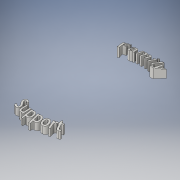
# Autodesk Inventor part: Team Pin Family-Text
Saved by Autodesk Inventor 2016 (Build 200138000, 138)
## iProperties
Created: 2016-02-20
Part Number: Team Pin Family-Text
Material: Generic
Document SubType Name: Modeling
Designer: RoksBot
Density: 1 g/cm^3
Appearance: White
Author: RoksBot
Autodesk Inventor part; units mm, degrees
ref_plane "YZ Plane" through (0, 0, 0) normal (1, 0, 0) x (0, 1, 0)
ref_plane "XZ Plane" through (0, 0, 0) normal (0, 1, 0) x (-1, 0, 0)
ref_plane "XY Plane" through (0, 0, 0) normal (0, 0, 1) x (1, 0, 0)
sketch "Sketch1" plane through (0, 0, 0) normal (0, 0, 1) x (1, 0, 0)
  line L0 (0, 0) -> (0, 8.6646) construction
  line L1 (20.9931, 1.27) -> (20.9931, 5.715)
  line L2 (20.9931, 5.715) -> (27.9781, 3.81)
  line L3 (27.9781, 3.81) -> (27.9781, 0)
  line L4 (27.9781, 0) -> (20.9931, 0)
  line L5 (20.9931, 1.27) -> (18.4531, 1.27)
  line L6 (18.4531, 1.27) -> (18.4531, 0)
  line L7 (18.4531, 0) -> (20.9931, 0)
  dimension "d0" = 20.9931
  dimension "d1" = 4.445
  dimension "d2" = 1.27
  dimension "d3" = 2.54
  dimension "d4" = 3.81
  dimension "d5" = 6.985
  constraints: 16 end point, 2 parallel, 2 perpendicular, 2 vertical, 1 horizontal, 1 horizontal alignment
  measures "d0" distance between parallel lines of L0 L1
  measures "d1" distance from line of L5 L1.end
  measures "d2" distance of L5.end L6.end
  measures "d3" distance between parallel lines of L1 L6
  measures "d4" distance of L2.end L3.end
  measures "d5" distance between parallel lines of L1 L3
revolve "Revolution1" add sketch "Sketch1" angle 360 about axis through (0, 0, 0) along (0, 1, 0)
sketch "Sketch2" plane through (0, 1.27, 0) normal (0, 1, 0) x (1, 0, 0)
  circle A0 centre (0, 0) radius 20.9931 projected
  circle A1 centre (0, 0) radius 27.9781 projected
  circle A2 centre (0, 0) radius 18.4531 projected
  circle A3 centre (0, 0) radius 20.9931 projected
  line L0 (-9.3205, 24.5047) -> (-8.9754, 23.5356)
  line L1 (-8.9754, 23.5356) -> (-7.525, 24.052)
  line L2 (-7.525, 24.052) -> (-7.3036, 23.43)
  line L3 (-7.3036, 23.43) -> (-8.754, 22.9135)
  line L4 (-8.754, 22.9135) -> (-8.0814, 21.0244)
  line L5 (-8.0814, 21.0244) -> (-8.8147, 20.7633)
  line L6 (-8.8147, 20.7633) -> (-10.2859, 24.8952)
  line L7 (-10.2859, 24.8952) -> (-7.5651, 25.8638)
  line L8 (-7.5651, 25.8638) -> (-7.3332, 25.2123)
  line L9 (-7.3332, 25.2123) -> (-9.3205, 24.5047)
  spline S0 degree 2 poles (-3.7722, 22.5301) (-3.8396, 22.3472) (-4.2977, 22.043) (-4.5708, 21.9904) knots 0 0 0 1 2 2 2
  spline S1 degree 2 poles (-4.5708, 21.9904) (-5.0792, 21.8924) (-5.7608, 22.2884) (-5.8502, 22.7525) knots 0 0 0 1 2 2 2
  spline S2 degree 2 poles (-5.8502, 22.7525) (-5.9554, 23.2985) (-5.2521, 24.0747) (-4.4979, 24.2201) knots 0 0 0 1 2 2 2
  spline S3 degree 2 poles (-4.4979, 24.2201) (-4.3682, 24.2451) (-4.1822, 24.2349) knots 0 0 0 1 1 1
  spline S4 degree 2 poles (-4.1822, 24.2349) (-4.2894, 24.7911) (-4.9924, 24.6557) knots 0 0 0 1 1 1
  spline S5 degree 2 poles (-4.9924, 24.6557) (-5.4087, 24.5754) (-5.6588, 24.3856) knots 0 0 0 1 1 1
  line L10 (-5.6588, 24.3856) -> (-5.9291, 24.9246)
  spline S6 degree 2 poles (-5.9291, 24.9246) (-5.5851, 25.1785) (-5.0596, 25.2798) knots 0 0 0 1 1 1
  spline S7 degree 2 poles (-5.0596, 25.2798) (-4.3395, 25.4186) (-3.5444, 24.8922) (-3.3688, 23.9811) knots 0 0 0 1 2 2 2
  line L11 (-3.3688, 23.9811) -> (-3.2386, 23.3054)
  spline S8 degree 2 poles (-3.2386, 23.3054) (-3.1176, 22.6775) (-2.8341, 22.5658) knots 0 0 0 1 1 1
  spline S9 degree 2 poles (-2.8341, 22.5658) (-2.896, 22.391) (-3.1033, 22.2732) (-3.2467, 22.2456) knots 0 0 0 1 2 2 2
  spline S10 degree 2 poles (-3.2467, 22.2456) (-3.4037, 22.2153) (-3.7016, 22.4021) (-3.7722, 22.5301) knots 0 0 0 1 2 2 2
  spline S11 degree 2 poles (-4.0682, 23.68) (-4.2631, 23.6813) (-4.3586, 23.6629) knots 0 0 0 1 1 1
  spline S12 degree 2 poles (-4.3586, 23.6629) (-5.2323, 23.4945) (-5.1231, 22.928) knots 0 0 0 1 1 1
  spline S13 degree 2 poles (-5.1231, 22.928) (-5.0415, 22.5049) (-4.5501, 22.5996) knots 0 0 0 1 1 1
  spline S14 degree 2 poles (-4.5501, 22.5996) (-3.8847, 22.7278) (-4.0116, 23.3865) knots 0 0 0 1 1 1
  line L12 (-4.0116, 23.3865) -> (-4.0682, 23.68)
  line L13 (1.4465, 22.5193) -> (1.4434, 24.5246)
  spline S15 degree 2 poles (1.4434, 24.5246) (1.4425, 25.1571) (0.876, 25.1563) knots 0 0 0 1 1 1
  spline S16 degree 2 poles (0.876, 25.1563) (0.7092, 25.156) (0.3967, 24.9574) (0.3343, 24.8288) knots 0 0 0 1 2 2 2
  line L14 (0.3343, 24.8288) -> (0.3378, 22.5176)
  line L15 (0.3378, 22.5176) -> (-0.4094, 22.5165)
  line L16 (-0.4094, 22.5165) -> (-0.4126, 24.64)
  spline S17 degree 2 poles (-0.4126, 24.64) (-0.4129, 24.8763) (-0.7053, 25.1539) (-0.9729, 25.1535) knots 0 0 0 1 2 2 2
  spline S18 degree 2 poles (-0.9729, 25.1535) (-1.1154, 25.1533) (-1.4452, 24.9442) (-1.5215, 24.819) knots 0 0 0 1 2 2 2
  line L17 (-1.5215, 24.819) -> (-1.518, 22.5148)
  line L18 (-1.518, 22.5148) -> (-2.2652, 22.5137)
  line L19 (-2.2652, 22.5137) -> (-2.2701, 25.718)
  line L20 (-2.2701, 25.718) -> (-1.7557, 25.7188)
  line L21 (-1.7557, 25.7188) -> (-1.6024, 25.4375)
  spline S19 degree 2 poles (-1.6024, 25.4375) (-1.2901, 25.7786) (-0.7966, 25.7793) knots 0 0 0 1 1 1
  spline S20 degree 2 poles (-0.7966, 25.7793) (-0.1606, 25.7803) (0.1631, 25.4332) knots 0 0 0 1 1 1
  spline S21 degree 2 poles (0.1631, 25.4332) (0.3054, 25.5933) (0.8056, 25.7817) (1.0593, 25.7821) knots 0 0 0 1 2 2 2
  spline S22 degree 2 poles (1.0593, 25.7821) (1.5945, 25.7829) (2.1897, 25.1721) (2.1905, 24.6369) knots 0 0 0 1 2 2 2
  line L22 (2.1905, 24.6369) -> (2.1937, 22.5204)
  line L23 (2.1937, 22.5204) -> (1.4465, 22.5193)
  line L24 (3.1822, 22.2932) -> (3.5833, 24.8512)
  line L25 (3.5833, 24.8512) -> (3.1781, 24.9147)
  line L26 (3.1781, 24.9147) -> (3.2734, 25.5224)
  line L27 (3.2734, 25.5224) -> (4.427, 25.3415)
  line L28 (4.427, 25.3415) -> (3.9307, 22.1759)
  line L29 (3.9307, 22.1759) -> (3.1822, 22.2932)
  spline S23 degree 2 poles (4.2524, 26.6283) (4.4309, 26.6003) (4.6423, 26.3103) (4.6143, 26.1318) knots 0 0 0 1 2 2 2
  spline S24 degree 2 poles (4.6143, 26.1318) (4.5863, 25.9533) (4.2963, 25.7419) (4.1178, 25.7699) knots 0 0 0 1 2 2 2
  spline S25 degree 2 poles (4.1178, 25.7699) (3.9393, 25.7979) (3.7279, 26.0879) (3.7559, 26.2664) knots 0 0 0 1 2 2 2
  spline S26 degree 2 poles (3.7559, 26.2664) (3.7839, 26.4449) (4.0739, 26.6563) (4.2524, 26.6283) knots 0 0 0 1 2 2 2
  line L30 (5.9373, 26.2566) -> (6.706, 26.2574)
  line L31 (6.706, 26.2574) -> (5.8627, 22.7535)
  spline S27 degree 2 poles (5.8627, 22.7535) (5.7244, 22.1791) (6.0422, 21.9847) knots 0 0 0 1 1 1
  spline S28 degree 2 poles (6.0422, 21.9847) (5.796, 21.7043) (5.3872, 21.8027) knots 0 0 0 1 1 1
  spline S29 degree 2 poles (5.3872, 21.8027) (4.8939, 21.9215) (5.0589, 22.6074) knots 0 0 0 1 1 1
  line L32 (5.0589, 22.6074) -> (5.9373, 26.2566)
  spline S30 degree 2 poles (7.6848, 20.6178) (7.4633, 20.3545) (6.5782, 20.2289) (6.085, 20.4083) knots 0 0 0 1 2 2 2
  line L33 (6.085, 20.4083) -> (6.3107, 21.0288)
  spline S31 degree 2 poles (6.3107, 21.0288) (7.1239, 20.7331) (7.2724, 21.1413) knots 0 0 0 1 1 1
  spline S32 degree 2 poles (7.2724, 21.1413) (7.371, 21.4124) (7.3475, 22.0496) knots 0 0 0 1 1 1
  line L34 (7.3475, 22.0496) -> (7.2541, 24.7314)
  line L35 (7.2541, 24.7314) -> (7.9824, 24.4665)
  line L36 (7.9824, 24.4665) -> (8.0554, 22.0843)
  line L37 (8.0554, 22.0843) -> (9.5567, 23.894)
  line L38 (9.5567, 23.894) -> (10.285, 23.6291)
  line L39 (10.285, 23.6291) -> (7.6848, 20.6178)
  line L40 (-10.2734, -23.3265) -> (-9.7699, -22.7922)
  spline S33 degree 2 poles (-9.7699, -22.7922) (-9.4653, -23.2443) (-9.0583, -23.3994) knots 0 0 0 1 1 1
  spline S34 degree 2 poles (-9.0583, -23.3994) (-8.4369, -23.6362) (-8.2709, -23.2009) knots 0 0 0 1 1 1
  spline S35 degree 2 poles (-8.2709, -23.2009) (-8.194, -22.9989) (-8.3467, -22.518) (-9.0861, -21.7088) (-9.2917, -21.2908) (-9.307, -20.8189) (-9.2132, -20.5728) knots 0 0 0 1 2 3 4 5 5 5
  spline S36 degree 2 poles (-9.2132, -20.5728) (-9.0376, -20.1123) (-8.1305, -19.7607) (-7.6005, -19.9627) knots 0 0 0 1 2 2 2
  spline S37 degree 2 poles (-7.6005, -19.9627) (-6.9096, -20.226) (-6.6864, -20.6073) knots 0 0 0 1 1 1
  line L41 (-6.6864, -20.6073) -> (-7.133, -21.1344)
  spline S38 degree 2 poles (-7.133, -21.1344) (-7.403, -20.7244) (-7.8131, -20.5681) knots 0 0 0 1 1 1
  spline S39 degree 2 poles (-7.8131, -20.5681) (-8.0592, -20.4743) (-8.426, -20.6308) (-8.5041, -20.8358) knots 0 0 0 1 2 2 2
  spline S40 degree 2 poles (-8.5041, -20.8358) (-8.6352, -21.1797) (-8.0187, -21.8374) knots 0 0 0 1 1 1
  spline S41 degree 2 poles (-8.0187, -21.8374) (-7.6926, -22.1856) (-7.4674, -22.6472) (-7.4472, -23.1535) (-7.5506, -23.4248) knots 0 0 0 1 2 3 3 3
  spline S42 degree 2 poles (-7.5506, -23.4248) (-7.7346, -23.9075) (-8.736, -24.2412) (-9.3765, -23.9971) knots 0 0 0 1 2 2 2
  spline S43 degree 2 poles (-9.3765, -23.9971) (-9.9349, -23.7843) (-10.2734, -23.3265) knots 0 0 0 1 1 1
  line L42 (-5.4016, -25.1294) -> (-5.3399, -24.8734)
  spline S44 degree 2 poles (-5.3399, -24.8734) (-5.5217, -24.965) (-6.0903, -25.0189) (-6.3102, -24.9659) knots 0 0 0 1 2 2 2
  spline S45 degree 2 poles (-6.3102, -24.9659) (-7.3638, -24.712) (-7.094, -23.5928) knots 0 0 0 1 1 1
  line L43 (-7.094, -23.5928) -> (-6.6208, -21.6301)
  line L44 (-6.6208, -21.6301) -> (-5.9152, -21.8002)
  line L45 (-5.9152, -21.8002) -> (-6.3757, -23.7104)
  spline S46 degree 2 poles (-6.3757, -23.7104) (-6.5157, -24.2913) (-5.9939, -24.4171) knots 0 0 0 1 1 1
  spline S47 degree 2 poles (-5.9939, -24.4171) (-5.751, -24.4756) (-5.2806, -24.3251) (-5.1721, -24.1776) knots 0 0 0 1 2 2 2
  line L46 (-5.1721, -24.1776) -> (-4.6713, -22.1001)
  line L47 (-4.6713, -22.1001) -> (-3.9657, -22.2702)
  line L48 (-3.9657, -22.2702) -> (-4.6959, -25.2995)
  line L49 (-4.6959, -25.2995) -> (-5.4016, -25.1294)
  line L50 (-3.2484, -25.4166) -> (-3.3791, -26.7098)
  line L51 (-3.3791, -26.7098) -> (-4.1013, -26.6368)
  line L52 (-4.1013, -26.6368) -> (-3.6652, -22.3239)
  line L53 (-3.6652, -22.3239) -> (-2.9431, -22.3969)
  line L54 (-2.9431, -22.3969) -> (-2.9641, -22.6052)
  spline S48 degree 2 poles (-2.9641, -22.6052) (-2.6652, -22.3673) (-2.2688, -22.4074) knots 0 0 0 1 1 1
  spline S49 degree 2 poles (-2.2688, -22.4074) (-0.7875, -22.5572) (-0.9523, -24.1862) knots 0 0 0 1 1 1
  spline S50 degree 2 poles (-0.9523, -24.1862) (-1.0293, -24.9487) (-1.9318, -25.6855) (-2.6405, -25.6138) knots 0 0 0 1 2 2 2
  spline S51 degree 2 poles (-2.6405, -25.6138) (-2.9798, -25.5795) (-3.2484, -25.4166) knots 0 0 0 1 1 1
  line L55 (-3.0198, -23.156) -> (-3.1842, -24.7818)
  spline S52 degree 2 poles (-3.1842, -24.7818) (-3.0019, -24.9597) (-2.74, -24.9862) knots 0 0 0 1 1 1
  spline S53 degree 2 poles (-2.74, -24.9862) (-2.2395, -25.0368) (-1.7546, -24.6039) (-1.7026, -24.09) knots 0 0 0 1 2 2 2
  spline S54 degree 2 poles (-1.7026, -24.09) (-1.6473, -23.5425) (-2.0354, -23.052) (-2.5359, -23.0014) knots 0 0 0 1 2 2 2
  spline S55 degree 2 poles (-2.5359, -23.0014) (-2.7979, -22.9749) (-3.0198, -23.156) knots 0 0 0 1 1 1
  line L56 (0.199, -25.6226) -> (0.2433, -26.9216)
  line L57 (0.2433, -26.9216) -> (-0.4821, -26.9464)
  line L58 (-0.4821, -26.9464) -> (-0.63, -22.614)
  line L59 (-0.63, -22.614) -> (0.0954, -22.5893)
  line L60 (0.0954, -22.5893) -> (0.1026, -22.7984)
  spline S56 degree 2 poles (0.1026, -22.7984) (0.3668, -22.5226) (0.7649, -22.509) knots 0 0 0 1 1 1
  spline S57 degree 2 poles (0.7649, -22.509) (2.2529, -22.4582) (2.3087, -24.0946) knots 0 0 0 1 1 1
  spline S58 degree 2 poles (2.3087, -24.0946) (2.3349, -24.8606) (1.5397, -25.7119) (0.8278, -25.7362) knots 0 0 0 1 2 2 2
  spline S59 degree 2 poles (0.8278, -25.7362) (0.487, -25.7479) (0.199, -25.6226) knots 0 0 0 1 1 1
  line L61 (0.1214, -23.3518) -> (0.1772, -24.9849)
  spline S60 degree 2 poles (0.1772, -24.9849) (0.3817, -25.1367) (0.6449, -25.1277) knots 0 0 0 1 1 1
  spline S61 degree 2 poles (0.6449, -25.1277) (1.1476, -25.1105) (1.5699, -24.6164) (1.5523, -24.1002) knots 0 0 0 1 2 2 2
  spline S62 degree 2 poles (1.5523, -24.1002) (1.5335, -23.5502) (1.0829, -23.1163) (0.5802, -23.1335) knots 0 0 0 1 2 2 2
  spline S63 degree 2 poles (0.5802, -23.1335) (0.317, -23.1424) (0.1214, -23.3518) knots 0 0 0 1 1 1
  spline S64 degree 2 poles (2.5369, -24.0418) (2.4185, -23.3394) (3.082, -22.3202) (3.7445, -22.2085) knots 0 0 0 1 2 2 2
  spline S65 degree 2 poles (3.7445, -22.2085) (4.447, -22.0901) (5.3624, -22.8088) (5.4865, -23.5445) knots 0 0 0 1 2 2 2
  spline S66 degree 2 poles (5.4865, -23.5445) (5.61, -24.2769) (4.9669, -25.2755) (4.2811, -25.3911) knots 0 0 0 1 2 2 2
  spline S67 degree 2 poles (4.2811, -25.3911) (3.582, -25.509) (2.6593, -24.7675) (2.5369, -24.0418) knots 0 0 0 1 2 2 2
  spline S68 degree 2 poles (3.2826, -23.9161) (3.4533, -24.9281) (4.1823, -24.8052) knots 0 0 0 1 1 1
  spline S69 degree 2 poles (4.1823, -24.8052) (4.5186, -24.7485) (4.8227, -24.1563) (4.7408, -23.6702) knots 0 0 0 1 2 2 2
  spline S70 degree 2 poles (4.7408, -23.6702) (4.5724, -22.6715) (3.8433, -22.7944) knots 0 0 0 1 1 1
  spline S71 degree 2 poles (3.8433, -22.7944) (3.5104, -22.8506) (3.2029, -23.4433) (3.2826, -23.9161) knots 0 0 0 1 2 2 2
  spline S72 degree 2 poles (7.3545, -22.0836) (7.1307, -22.0149) (6.9069, -22.0797) knots 0 0 0 1 1 1
  spline S73 degree 2 poles (6.9069, -22.0797) (6.6637, -22.1502) (6.4154, -22.7002) (6.5074, -23.018) knots 0 0 0 1 2 2 2
  line L62 (6.5074, -23.018) -> (7.0007, -24.7204)
  line L63 (7.0007, -24.7204) -> (6.3035, -24.9224)
  line L64 (6.3035, -24.9224) -> (5.4373, -21.9326)
  line L65 (5.4373, -21.9326) -> (6.1344, -21.7306)
  line L66 (6.1344, -21.7306) -> (6.2143, -22.0063)
  spline S74 degree 2 poles (6.2143, -22.0063) (6.4103, -21.5909) (6.8967, -21.45) knots 0 0 0 1 1 1
  spline S75 degree 2 poles (6.8967, -21.45) (7.2534, -21.3467) (7.4767, -21.4015) knots 0 0 0 1 1 1
  line L67 (7.4767, -21.4015) -> (7.3545, -22.0836)
  line L68 (7.9067, -21.7827) -> (7.5709, -21.9158)
  line L69 (7.5709, -21.9158) -> (7.3557, -21.3729)
  line L70 (7.3557, -21.3729) -> (7.6915, -21.2397)
  line L71 (7.6915, -21.2397) -> (7.4576, -20.6497)
  line L72 (7.4576, -20.6497) -> (8.0341, -20.1343)
  line L73 (8.0341, -20.1343) -> (8.3662, -20.9723)
  line L74 (8.3662, -20.9723) -> (9.1603, -20.6575)
  line L75 (9.1603, -20.6575) -> (9.3755, -21.2005)
  line L76 (9.3755, -21.2005) -> (8.5815, -21.5152)
  line L77 (8.5815, -21.5152) -> (9.0829, -22.78)
  spline S76 degree 2 poles (9.0829, -22.78) (9.206, -23.0907) (9.5026, -23.271) (9.7443, -23.1752) knots 0 0 0 1 2 2 2
  spline S77 degree 2 poles (9.7443, -23.1752) (9.9891, -23.0781) (10.1471, -22.8629) knots 0 0 0 1 1 1
  line L78 (10.1471, -22.8629) -> (10.3935, -23.4844)
  spline S78 degree 2 poles (10.3935, -23.4844) (10.1904, -23.6593) (9.7573, -23.831) knots 0 0 0 1 1 1
  spline S79 degree 2 poles (9.7573, -23.831) (9.3242, -24.0027) (8.6656, -23.6972) (8.4865, -23.2452) knots 0 0 0 1 2 2 2
  line L79 (8.4865, -23.2452) -> (7.9067, -21.7827)
  constraints: 2 other
extrude "Extrusion1" cut sketch "Sketch2" along normal through all contours L0 L1 L2 L3 L4 L5 L6 L7 L8 L9 | S0 S1 S2 S3 S4 S5 L10 S6 S7 L11 S8 S9 S10 | L13 S15 S16 L14 L15 L16 S17 S18 L17 L18 L19 L20 L21 S19 S20 S21 S22 L22 L23 | L24 L25 L26 L27 L28 L29 | S23 S24 S25 S26 | L30 L31 S27 S28 S29 L32 | S30 L33 S31 S32 L34 L35 L36 L37 L38 L39 | L40 S33 S34 S35 S36 S37 L41 S38 S39 S40 S41 S42 S43 | L42 S44 S45 L43 L44 L45 S46 S47 L46 L47 L48 L49 | L50 L51 L52 L53 L54 S48 S49 S50 S51 | L56 L57 L58 L59 L60 S56 S57 S58 S59 | S64 S65 S66 S67 | S72 S73 L62 L63 L64 L65 L66 S74 S75 L69 L67 | L69 S75 L67 | L67 S75 L69 L70 L71 L72 L73 L74 L75 L76 L77 S76 S77 L78 S78 S79 L79 L68 keep common part
body "Solid1"
